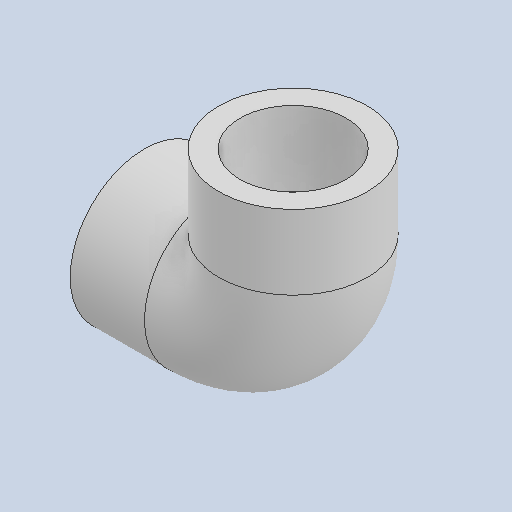
# Autodesk Inventor part: Knee
Saved by Autodesk Inventor 2025 (Build 290162000, 162)
## iProperties
Created: 2025-07-16
Part Number: Knee
Material: Generic
Document SubType Name: Modeling
Designer: Pravoslav
Density: 1 g/cm^3
Appearance: Default
Author: Pravoslav
Autodesk Inventor part; units mm, degrees
ref_plane "YZ Plane" through (0, 0, 0) normal (1, 0, 0) x (0, 1, 0)
ref_plane "XY Plane" through (0, 0, 0) normal (0, 0, 1) x (1, 0, 0)
sketch "Sketch1" plane through (0, 0, 0) normal (0, 1, 0) x (-1, 0, 0)
  circle A0 centre (0, 0) radius 5
  circle A1 centre (0, 0) radius 3.575
  line L0 (5, 0) -> (5, -7.589)
  dimension "d0" = 10
  dimension "d1" = 7.15
  constraints: 2 coincident, 2 end point, 2 vertical, 1 centre point, 1 horizontal alignment, 2 other
  measures "d1" diameter of A1
revolve "Revolution1" add sketch "Sketch1" angle 90 about axis through (-5, 0, 0) along (0, 0, -1)
sketch "Sketch3" plane through (-5, -5, 0) normal (-1, 0, 0) x (0, 0, 1)
  circle A0 centre (0, 0) radius 3.575
  circle A1 centre (0, 0) radius 5
  point P0 (0, 5)
  dimension "d8" = 7.15
  dimension "d9" = 10
  constraints: 2 centre point, 1 coincident
  measures "d8" diameter of A0
  measures "d9" diameter of A1
extrude "Extrusion1" add sketch "Sketch3" along normal blind 5
sketch "Sketch4" plane through (0, 0, 0) normal (0, 1, 0) x (1, 0, 0)
  circle A0 centre (0, 0) radius 3.575
  circle A1 centre (0, 0) radius 5
  dimension "d12" = 7.15
  dimension "d13" = 10
  dimension "d4" = 10
  dimension "d5" = 5
  dimension "d6" = 7.15
  constraints: 2 centre point, 2 coincident
  measures "d12" diameter of A0
  measures "d13" diameter of A1
extrude "Extrusion2" add sketch "Sketch4" along normal blind 5
ref_plane "Work Plane1" through (0, 0, 0) normal (0, 0, 1) x (1, 0, 0)
body "Solid1"
